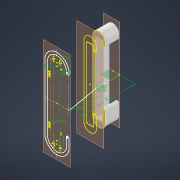
# Autodesk Inventor part: Top Part
Saved by Autodesk Inventor 2021.3 (Build 253353000, 353)
## iProperties
Created: 2021-07-04
Part Number: Top Part
Material: Generic
Document SubType Name: Modeling
Designer: trl121
Density: 1 g/cm^3
Appearance: Default
Author: trl121
Autodesk Inventor part; units mm, degrees
ref_plane "YZ Plane" through (0, 0, 0) normal (1, 0, 0) x (0, 1, 0)
ref_plane "XZ Plane" through (0, 0, 0) normal (0, 1, 0) x (-1, 0, 0)
ref_plane "XY Plane" through (0, 0, 0) normal (0, 0, 1) x (1, 0, 0)
ref_plane "Work Plane12" through (0, 0, 0) normal (0, 0, 1) x (1, 0, 0)
sketch "Sketch13" plane through (0, 0, 0) normal (0, 0, 1) x (1, 0, 0)
  line L0 (18.0369, 91.6315) -> (18.0369, 101.4813) projected
  arc A0 (12.9569, 86.5515) -> (18.0369, 91.6315) centre (12.9569, 91.6315) ccw projected
  arc A1 (10.4169, 87.8215) -> (11.6869, 86.5515) centre (11.6869, 87.8215) ccw projected
  line L1 (11.6869, 86.5515) -> (12.9569, 86.5515) projected
  line L2 (10.4169, 100.2113) -> (10.4169, 87.8215) projected
  arc A2 (18.0369, 101.4813) -> (-18.0369, 101.4813) centre (0, 101.4813) ccw projected
  arc A3 (10.4169, 100.2113) -> (9.1469, 101.4813) centre (9.1469, 100.2113) ccw projected
  line L3 (-9.1469, 101.4813) -> (9.1469, 101.4813) projected
  arc A4 (-9.1469, 101.4813) -> (-10.4169, 100.2113) centre (-9.1469, 100.2113) ccw projected
  line L4 (-10.4169, -100.2113) -> (-10.4169, 100.2113) projected
  line L5 (-18.0369, 101.4813) -> (-18.0369, 69.971) projected
  line L6 (-18.0369, 57.029) -> (-18.0369, -57.029) projected
  line L7 (-18.0369, -69.971) -> (-18.0369, -101.4813) projected
  arc A5 (-18.0369, -101.4813) -> (18.0369, -101.4813) centre (0, -101.4813) ccw projected
  line L8 (18.0369, -101.4813) -> (18.0369, -70.9285) projected
  arc A6 (18.0369, -70.9285) -> (12.9569, -65.8485) centre (12.9569, -70.9285) ccw projected
  line L9 (12.9569, -65.8485) -> (11.6869, -65.8485) projected
  arc A7 (11.6869, -65.8485) -> (10.4169, -67.1185) centre (11.6869, -67.1185) ccw projected
  line L10 (10.4169, -67.1185) -> (10.4169, -100.2113) projected
  arc A8 (9.1469, -101.4813) -> (10.4169, -100.2113) centre (9.1469, -100.2113) ccw projected
  line L11 (9.1469, -101.4813) -> (-9.1469, -101.4813) projected
  arc A9 (-10.4169, -100.2113) -> (-9.1469, -101.4813) centre (-9.1469, -100.2113) ccw projected
  line L12 (-18.0369, 69.971) -> (-18.0369, 57.029)
  line L13 (-18.0369, -57.029) -> (-18.0369, -69.971)
  line L14 (18.0369, 91.6315) -> (18.0369, -70.9285) construction
  point P0 (0, 0)
  constraints: 6 end point, 2 vertical, 1 collinear, 1 tangent
ref_plane "Work Plane4" through (-9.1469, 0, 0) normal (0, -1, 0) x (1, 0, 0)
sketch "Loft Sketch" plane through (-9.1469, 0, 0) normal (0, -1, 0) x (1, 0, 0)
  line L0 (27.1839, 65.45) -> (43.979, 160.7)
  line L1 (27.1839, 65.45) -> (27.1839, 40.05)
  point P0 (9.1469, 0)
  point P1 (27.1839, 0)
  point P2 (27.1839, 0)
  point P3 (27.1839, 0)
  dimension "d6" = 170
  dimension "d7" = 95.25
  dimension "d65" = 25.4
  dimension "d68" = 160.7
  constraints: 4 end point, 1 vertical, 1 vertical alignment
  measures "d6" angle of L0 L1
  measures "d7" vertical distance of L0.end L0.start
  measures "d65" distance of L0.start L1.end
  measures "d68" vertical distance of L0.end point (27.184, 0)
extrude "Extrusion6" add sketch "Sketch13" along normal up to surface (40.05 mm away)
sketch "Lower" plane through (0, 101.4813, 40.05) normal (0, 0, 1) x (1, 0, 0)
  line L0 (10.4169, -13.6598) -> (10.4169, -1.27) projected
  arc A0 (10.4169, -13.6598) -> (11.6869, -14.9298) centre (11.6869, -13.6598) ccw projected
  line L1 (12.9569, -14.9298) -> (11.6869, -14.9298) projected
  arc A1 (12.9569, -14.9298) -> (18.0369, -9.8498) centre (12.9569, -9.8498) ccw projected
  line L2 (18.0369, 0) -> (18.0369, -9.8498) projected
  arc A2 (18.0369, 0) -> (-18.0369, 0) centre (0, 0) ccw projected
  line L3 (-18.0369, -202.9627) -> (-18.0369, 0) projected
  arc A3 (-18.0369, -202.9627) -> (18.0369, -202.9627) centre (0, -202.9627) ccw projected
  line L4 (18.0369, -172.4098) -> (18.0369, -202.9627) projected
  arc A4 (18.0369, -172.4098) -> (12.9569, -167.3298) centre (12.9569, -172.4098) ccw projected
  line L5 (11.6869, -167.3298) -> (12.9569, -167.3298) projected
  arc A5 (11.6869, -167.3298) -> (10.4169, -168.5998) centre (11.6869, -168.5998) ccw projected
  line L6 (10.4169, -201.6927) -> (10.4169, -168.5998) projected
  arc A6 (9.1469, -202.9627) -> (10.4169, -201.6927) centre (9.1469, -201.6927) ccw projected
  line L7 (-9.1469, -202.9627) -> (9.1469, -202.9627) projected
  arc A7 (-10.4169, -201.6927) -> (-9.1469, -202.9627) centre (-9.1469, -201.6927) ccw projected
  line L8 (-10.4169, -1.27) -> (-10.4169, -201.6927) projected
  arc A8 (-9.1469, 0) -> (-10.4169, -1.27) centre (-9.1469, -1.27) ccw projected
  line L9 (9.1469, 0) -> (-9.1469, 0) projected
  arc A9 (10.4169, -1.27) -> (9.1469, 0) centre (9.1469, -1.27) ccw projected
  point P0 (0, -101.4813)
ref_plane "Mid Lof Plane" through (18.0369, 0, 65.45) normal (0, 0, 1) x (1, 0, 0)
sketch "Mid" plane through (18.0369, 0, 65.45) normal (0, 0, 1) x (1, 0, 0)
  line L0 (-7.62, 87.8215) -> (-7.62, 100.2113) projected
  arc A0 (-7.62, 87.8215) -> (-6.35, 86.5515) centre (-6.35, 87.8215) ccw projected
  line L1 (-5.08, 86.5515) -> (-6.35, 86.5515) projected
  arc A1 (-5.08, 86.5515) -> (0, 91.6315) centre (-5.08, 91.6315) ccw projected
  line L2 (0, 101.4813) -> (0, 91.6315) projected
  arc A2 (0, 101.4813) -> (-36.0739, 101.4813) centre (-18.0369, 101.4813) ccw projected
  line L3 (-36.0739, -101.4813) -> (-36.0739, 101.4813) projected
  arc A3 (-36.0739, -101.4813) -> (0, -101.4813) centre (-18.0369, -101.4813) ccw projected
  line L4 (0, -70.9285) -> (0, -101.4813) projected
  arc A4 (0, -70.9285) -> (-5.08, -65.8485) centre (-5.08, -70.9285) ccw projected
  line L5 (-6.35, -65.8485) -> (-5.08, -65.8485) projected
  arc A5 (-6.35, -65.8485) -> (-7.62, -67.1185) centre (-6.35, -67.1185) ccw projected
  line L6 (-7.62, -100.2113) -> (-7.62, -67.1185) projected
  arc A6 (-8.89, -101.4813) -> (-7.62, -100.2113) centre (-8.89, -100.2113) ccw projected
  line L7 (-27.1839, -101.4813) -> (-8.89, -101.4813) projected
  arc A7 (-28.4539, -100.2113) -> (-27.1839, -101.4813) centre (-27.1839, -100.2113) ccw projected
  line L8 (-28.4539, 100.2113) -> (-28.4539, -100.2113) projected
  arc A8 (-27.1839, 101.4813) -> (-28.4539, 100.2113) centre (-27.1839, 100.2113) ccw projected
  line L9 (-8.89, 101.4813) -> (-27.1839, 101.4813) projected
  arc A9 (-7.62, 100.2113) -> (-8.89, 101.4813) centre (-8.89, 100.2113) ccw projected
  point P0 (-18.0369, 0)
ref_plane "Work Plane5" through (34.8321, 0, 160.7) normal (0, 0, 1) x (1, 0, 0)
ref_plane "Work Plane7" through (0, 0, 0) normal (0, 0, 1) x (1, 0, 0)
sketch "Sketch6" plane through (34.8321, 0, 160.7) normal (0, 0, 1) x (1, 0, 0)
  line L0 (0, 92.3062) -> (0, 91.6315)
  line L1 (-62.0442, 92.3062) -> (-62.0442, 0)
  line L2 (-69.6642, 0) -> (-69.6642, 92.3062)
  line L3 (0, 91.6315) -> (0, 0) construction
  line L4 (-52.869, 0) -> (-45.249, 0) construction
  arc A0 (-34.8321, 119.5183) -> (-62.0442, 92.3062) centre (-34.8321, 92.3062) ccw
  arc A1 (-7.62, 92.3062) -> (-34.8321, 119.5183) centre (-34.8321, 92.3062) ccw
  line L5 (-7.62, 92.3062) -> (-7.62, 89.0915)
  arc A2 (-7.62, 89.0915) -> (-5.08, 86.5515) centre (-5.08, 89.0915) ccw
  line L6 (-5.08, 86.5515) -> (-5.08, 86.5515)
  arc A3 (-5.08, 86.5515) -> (0, 91.6315) centre (-5.08, 91.6315) ccw
  line L7 (-7.62, 90.6989) -> (0, 90.6989) construction
  line L8 (-69.6642, 0) -> (-62.0442, 0) construction
  arc A4 (0, 92.3062) -> (-69.6642, 92.3062) centre (-34.8321, 92.3062) ccw
  line L9 (0, 0) -> (-69.6642, 0) construction
  line L10 (0, -92.3062) -> (0, -70.9285)
  line L11 (-62.0442, -92.3062) -> (-62.0442, 0)
  line L12 (-69.6642, 0) -> (-69.6642, -92.3062)
  arc A5 (-62.0442, -92.3062) -> (-34.8321, -119.5183) centre (-34.8321, -92.3062) ccw
  arc A6 (-34.8321, -119.5183) -> (-7.62, -92.3062) centre (-34.8321, -92.3062) ccw
  line L13 (-7.62, -92.3062) -> (-7.62, -68.3885)
  arc A7 (-5.08, -65.8485) -> (-7.62, -68.3885) centre (-5.08, -68.3885) ccw
  line L14 (-5.08, -65.8485) -> (-5.08, -65.8485)
  arc A8 (0, -70.9285) -> (-5.08, -65.8485) centre (-5.08, -70.9285) ccw
  arc A9 (-69.6642, -92.3062) -> (0, -92.3062) centre (-34.8321, -92.3062) ccw
  arc A10 (-57.314, -56.6624) -> (-59.219, -57.7622) centre (-57.949, -57.7622) ccw construction
  line L15 (-59.219, -57.7622) -> (-59.219, -69.2378) construction
  arc A11 (-59.219, -69.2378) -> (-57.314, -70.3376) centre (-57.949, -69.2378) ccw construction
  line L16 (-57.314, -70.3376) -> (-54.774, -68.8712) construction
  arc A12 (-52.869, -69.971) -> (-54.774, -68.8712) centre (-54.139, -69.971) ccw construction
  line L17 (-52.869, -69.971) -> (-52.869, -101.4813) construction
  arc A13 (-52.869, -101.4813) -> (-16.7951, -101.4813) centre (-34.8321, -101.4813) ccw construction
  line L18 (-16.7951, -101.4813) -> (-16.7951, -70.9285) construction
  arc A14 (-16.7951, -70.9285) -> (-21.8751, -65.8485) centre (-21.8751, -70.9285) ccw construction
  line L19 (-21.8751, -65.8485) -> (-23.1451, -65.8485) construction
  arc A15 (-23.1451, -65.8485) -> (-24.4151, -67.1185) centre (-23.1451, -67.1185) ccw construction
  line L20 (-24.4151, -67.1185) -> (-24.4151, -100.2113) construction
  arc A16 (-25.6851, -101.4813) -> (-24.4151, -100.2113) centre (-25.6851, -100.2113) ccw construction
  line L21 (-25.6851, -101.4813) -> (-43.979, -101.4813) construction
  arc A17 (-45.249, -100.2113) -> (-43.979, -101.4813) centre (-43.979, -100.2113) ccw construction
  line L22 (-45.249, -100.2113) -> (-45.249, 100.2113) construction
  arc A18 (-43.979, 101.4813) -> (-45.249, 100.2113) centre (-43.979, 100.2113) ccw construction
  line L23 (-43.979, 101.4813) -> (-25.6851, 101.4813) construction
  arc A19 (-24.4151, 100.2113) -> (-25.6851, 101.4813) centre (-25.6851, 100.2113) ccw construction
  line L24 (-24.4151, 100.2113) -> (-24.4151, 87.8215) construction
  arc A20 (-24.4151, 87.8215) -> (-23.1451, 86.5515) centre (-23.1451, 87.8215) ccw construction
  line L25 (-23.1451, 86.5515) -> (-21.8751, 86.5515) construction
  arc A21 (-21.8751, 86.5515) -> (-16.7951, 91.6315) centre (-21.8751, 91.6315) ccw construction
  line L26 (-16.7951, 91.6315) -> (-16.7951, 101.4813) construction
  arc A22 (-16.7951, 101.4813) -> (-52.869, 101.4813) centre (-34.8321, 101.4813) ccw construction
  line L27 (-52.869, 101.4813) -> (-52.869, 69.971) construction
  arc A23 (-54.774, 68.8712) -> (-52.869, 69.971) centre (-54.139, 69.971) ccw construction
  line L28 (-54.774, 68.8712) -> (-57.314, 70.3376) construction
  arc A24 (-57.314, 70.3376) -> (-59.219, 69.2378) centre (-57.949, 69.2378) ccw construction
  line L29 (-59.219, 69.2378) -> (-59.219, 57.7622) construction
  arc A25 (-59.219, 57.7622) -> (-57.314, 56.6624) centre (-57.949, 57.7622) ccw construction
  line L30 (-57.314, 56.6624) -> (-54.774, 58.1288) construction
  arc A26 (-52.869, 57.029) -> (-54.774, 58.1288) centre (-54.139, 57.029) ccw construction
  line L31 (-52.869, 57.029) -> (-52.869, -57.029) construction
  arc A27 (-54.774, -58.1288) -> (-52.869, -57.029) centre (-54.139, -57.029) ccw construction
  line L32 (-54.774, -58.1288) -> (-57.314, -56.6624) construction
  line L33 (-42.4521, 102.7513) -> (-42.4521, 105.2913) construction
  arc A28 (-43.7221, 104.0213) -> (-42.4521, 105.2913) centre (-43.7221, 105.2913) ccw construction
  line L34 (-43.7221, 104.0213) -> (-47.5321, 104.0213) construction
  arc A29 (-48.8021, 105.2913) -> (-47.5321, 104.0213) centre (-47.5321, 105.2913) ccw construction
  line L35 (-48.8021, 105.2913) -> (-48.8021, 107.8313) construction
  arc A30 (-44.0396, 113.9797) -> (-48.8021, 107.8313) centre (-42.4521, 107.8313) ccw construction
  arc A31 (-42.4521, 112.75) -> (-44.0396, 113.9797) centre (-43.7221, 112.75) ccw construction
  line L36 (-42.4521, 112.75) -> (-42.4521, 109.1013) construction
  line L37 (-42.4521, 109.1013) -> (-27.2121, 109.1013) construction
  line L38 (-27.2121, 109.1013) -> (-27.2121, 112.75) construction
  arc A32 (-25.6246, 113.9797) -> (-27.2121, 112.75) centre (-25.9421, 112.75) ccw construction
  arc A33 (-20.8621, 107.8313) -> (-25.6246, 113.9797) centre (-27.2121, 107.8313) ccw construction
  line L39 (-20.8621, 107.8313) -> (-20.8621, 105.2913) construction
  arc A34 (-22.1321, 104.0213) -> (-20.8621, 105.2913) centre (-22.1321, 105.2913) ccw construction
  line L40 (-22.1321, 104.0213) -> (-25.9421, 104.0213) construction
  arc A35 (-27.2121, 105.2913) -> (-25.9421, 104.0213) centre (-25.9421, 105.2913) ccw construction
  line L41 (-27.2121, 105.2913) -> (-27.2121, 102.7513) construction
  line L42 (-27.2121, 102.7513) -> (-42.4521, 102.7513) construction
  line L43 (-27.2121, -109.1013) -> (-42.4521, -109.1013) construction
  line L44 (-42.4521, -109.1013) -> (-42.4521, -112.75) construction
  arc A36 (-44.0396, -113.9797) -> (-42.4521, -112.75) centre (-43.7221, -112.75) ccw construction
  arc A37 (-48.8021, -107.8313) -> (-44.0396, -113.9797) centre (-42.4521, -107.8313) ccw construction
  line L45 (-48.8021, -107.8313) -> (-48.8021, -105.2913) construction
  arc A38 (-47.5321, -104.0213) -> (-48.8021, -105.2913) centre (-47.5321, -105.2913) ccw construction
  line L46 (-47.5321, -104.0213) -> (-43.7221, -104.0213) construction
  arc A39 (-42.4521, -105.2913) -> (-43.7221, -104.0213) centre (-43.7221, -105.2913) ccw construction
  line L47 (-42.4521, -105.2913) -> (-42.4521, -102.7513) construction
  line L48 (-42.4521, -102.7513) -> (-27.2121, -102.7513) construction
  line L49 (-27.2121, -102.7513) -> (-27.2121, -105.2913) construction
  arc A40 (-25.9421, -104.0213) -> (-27.2121, -105.2913) centre (-25.9421, -105.2913) ccw construction
  line L50 (-25.9421, -104.0213) -> (-22.1321, -104.0213) construction
  arc A41 (-20.8621, -105.2913) -> (-22.1321, -104.0213) centre (-22.1321, -105.2913) ccw construction
  line L51 (-20.8621, -105.2913) -> (-20.8621, -107.8313) construction
  arc A42 (-25.6246, -113.9797) -> (-20.8621, -107.8313) centre (-27.2121, -107.8313) ccw construction
  arc A43 (-27.2121, -112.75) -> (-25.6246, -113.9797) centre (-25.9421, -112.75) ccw construction
  line L52 (-27.2121, -112.75) -> (-27.2121, -109.1013) construction
  line L53 (-24.4151, 94.0164) -> (-16.7951, 94.0164) construction
  line L54 (-45.249, 100.2113) -> (-52.869, 100.2113) construction
  line L55 (-62.0442, 92.3062) -> (-69.6642, 92.3062) construction
  line L56 (-57.949, -65.405) -> (-57.949, -61.595) projected
  arc A44 (-56.679, -60.325) -> (-57.949, -61.595) centre (-56.679, -61.595) ccw projected
  line L57 (-56.679, -60.325) -> (-55.409, -60.325) projected
  arc A45 (-54.139, -61.595) -> (-55.409, -60.325) centre (-55.409, -61.595) ccw projected
  line L58 (-54.139, -61.595) -> (-54.139, -65.405) projected
  arc A46 (-55.409, -66.675) -> (-54.139, -65.405) centre (-55.409, -65.405) ccw projected
  line L59 (-55.409, -66.675) -> (-56.679, -66.675) projected
  arc A47 (-57.949, -65.405) -> (-56.679, -66.675) centre (-56.679, -65.405) ccw projected
  line L60 (-57.949, 61.595) -> (-57.949, 65.405) projected
  arc A48 (-56.679, 66.675) -> (-57.949, 65.405) centre (-56.679, 65.405) ccw projected
  line L61 (-56.679, 66.675) -> (-55.409, 66.675) projected
  arc A49 (-54.139, 65.405) -> (-55.409, 66.675) centre (-55.409, 65.405) ccw projected
  line L62 (-54.139, 65.405) -> (-54.139, 61.595) projected
  arc A50 (-55.409, 60.325) -> (-54.139, 61.595) centre (-55.409, 61.595) ccw projected
  line L63 (-55.409, 60.325) -> (-56.679, 60.325) projected
  arc A51 (-57.949, 61.595) -> (-56.679, 60.325) centre (-56.679, 61.595) ccw projected
  point P0 (-34.8321, 0)
  point P1 (-34.8321, 127.1383)
  point P2 (-34.8321, -127.1383)
  dimension "d25" = 27.2121
  dimension "d26" = 27.2121
  dimension "d29" = 1.27
  dimension "d30" = 202.9627
  dimension "d31" = 9.1751
  constraints: 37 end point, 24 point on circle, 13 tangent, 10 centre point, 9 symmetric about line, 6 vertical, 5 perpendicular, 4 equal radius, 4 point on line, 3 collinear, 2 coincident, 2 horizontal, 2 midpoint, 2 parallel, 1 horizontal alignment, 5 other
  measures "d25" distance from line of L5 A22.centre
  measures "d26" distance from line of L1 A22.centre
  measures "d29" radius of A19
  measures "d30" distance between parallel lines of L21 L23
  measures "d31" distance between parallel lines of L5 L26
sketch "Sketch8" plane through (0, 101.4813, 0) normal (0, 0, -1) x (-1, 0, 0)
  arc A0 (19.9419, -170.3525) -> (18.0369, -171.4524) centre (19.3069, -171.4524) ccw projected
  line L0 (22.4819, -171.819) -> (19.9419, -170.3525) projected
  arc A1 (22.4819, -171.819) -> (24.3869, -170.7191) centre (23.1169, -170.7191) ccw projected
  line L1 (24.3869, -159.2435) -> (24.3869, -170.7191) projected
  arc A2 (24.3869, -159.2435) -> (22.4819, -158.1437) centre (23.1169, -159.2435) ccw projected
  line L2 (19.9419, -159.6102) -> (22.4819, -158.1437) projected
  arc A3 (18.0369, -158.5103) -> (19.9419, -159.6102) centre (19.3069, -158.5103) ccw projected
  line L3 (19.9419, -32.6102) -> (22.4819, -31.1437) projected
  arc A4 (18.0369, -31.5103) -> (19.9419, -32.6102) centre (19.3069, -31.5103) ccw projected
  arc A5 (24.3869, -32.2435) -> (22.4819, -31.1437) centre (23.1169, -32.2435) ccw projected
  line L4 (24.3869, -32.2435) -> (24.3869, -43.7191) projected
  arc A6 (19.9419, -43.3525) -> (18.0369, -44.4524) centre (19.3069, -44.4524) ccw projected
  line L5 (22.4819, -44.819) -> (19.9419, -43.3525) projected
  arc A7 (22.4819, -44.819) -> (24.3869, -43.7191) centre (23.1169, -43.7191) ccw projected
  line L6 (18.0369, -31.5103) -> (18.0369, -44.4524)
  line L7 (18.0369, 0) -> (18.0369, -202.9627) construction
  line L8 (18.0369, -171.4524) -> (18.0369, -158.5103)
  point P0 (0, -101.4813)
  constraints: 4 end point, 2 collinear
sketch "Sketch9" plane through (0, 101.4813, 0) normal (0, 0, -1) x (-1, 0, 0)
  line L0 (7.62, 7.62) -> (-7.62, 7.62) construction
  line L1 (7.62, 11.2687) -> (7.62, 7.62) construction
  arc A0 (9.2075, 12.4984) -> (7.62, 11.2687) centre (8.89, 11.2687) ccw construction
  arc A1 (13.97, 6.35) -> (9.2075, 12.4984) centre (7.62, 6.35) ccw construction
  line L2 (13.97, 3.81) -> (13.97, 6.35) construction
  arc A2 (12.7, 2.54) -> (13.97, 3.81) centre (12.7, 3.81) ccw construction
  line L3 (8.89, 2.54) -> (12.7, 2.54) construction
  line L4 (7.62, 1.27) -> (7.62, 3.81) construction
  line L5 (-7.62, 7.62) -> (-7.62, 11.2687) construction
  arc A3 (-7.62, 11.2687) -> (-9.2075, 12.4984) centre (-8.89, 11.2687) ccw construction
  arc A4 (-9.2075, 12.4984) -> (-13.97, 6.35) centre (-7.62, 6.35) ccw construction
  line L6 (-13.97, 6.35) -> (-13.97, 3.81) construction
  arc A5 (-13.97, 3.81) -> (-12.7, 2.54) centre (-12.7, 3.81) ccw construction
  line L7 (-12.7, 2.54) -> (-8.89, 2.54) construction
  line L8 (-7.62, 3.81) -> (-7.62, 1.27) construction
  line L9 (-7.62, 1.27) -> (7.62, 1.27) construction
  line L10 (-7.874, 2.286) -> (-12.7, 2.286)
  arc A6 (-14.224, 3.81) -> (-12.7, 2.286) centre (-12.7, 3.81) ccw
  line L11 (-14.224, 3.81) -> (-14.224, 6.35)
  arc A7 (-9.271, 12.7443) -> (-14.224, 6.35) centre (-7.62, 6.35) ccw
  arc A8 (-7.366, 11.2687) -> (-9.271, 12.7443) centre (-8.89, 11.2687) ccw
  line L12 (-7.366, 11.2687) -> (-7.366, 6.35)
  line L13 (7.366, 6.35) -> (7.366, 11.2687)
  arc A9 (9.271, 12.7443) -> (7.366, 11.2687) centre (8.89, 11.2687) ccw
  arc A10 (14.224, 6.35) -> (9.271, 12.7443) centre (7.62, 6.35) ccw
  line L14 (14.224, 6.35) -> (14.224, 3.81)
  arc A11 (12.7, 2.286) -> (14.224, 3.81) centre (12.7, 3.81) ccw
  line L15 (12.7, 2.286) -> (7.874, 2.286)
  line L16 (7.874, 2.286) -> (7.874, -0.254)
  line L17 (-7.874, -0.254) -> (-7.874, 2.286)
  line L18 (7.874, -0.254) -> (-7.874, -0.254)
  line L19 (9.1469, 0) -> (-9.1469, 0) construction
  line L20 (7.366, 6.35) -> (-7.366, 6.35)
  point P0 (0, -101.4813)
  dimension "d45" = 0.254
  dimension "d46" = 0.254
  dimension "d47" = 0.254
  dimension "d50" = 0.254
  dimension "d51" = 0.254
  dimension "d52" = 1.27
  constraints: 20 end point, 12 point on circle, 6 centre point, 1 horizontal, 1 parallel, 10 other
  measures "d45" distance between parallel lines of L16 L4
  measures "d46" distance between parallel lines of L8 L17
  measures "d47" distance between parallel lines of L18 L19
  measures "d50" distance between parallel lines of L13 L1
  measures "d51" distance between parallel lines of L12 L5
  measures "d52" distance between parallel lines of L0 L20
sketch "Sketch10" plane through (-7.366, 109.3553, 0) normal (-1, 0, 0) x (0, 0, 1)
  line L0 (-12.7, -1.016) -> (7.62, -1.524) construction
  line L1 (7.62, 1.016) -> (7.62, -1.524) construction
  line L2 (11.8332, -1.7226) -> (7.62, 1.016) construction
  line L3 (12.2002, -1.7226) -> (12.2002, -1.9766)
  line L4 (12.2002, -1.9766) -> (0, -1.9766)
  line L5 (0, -4.064) -> (0, -1.524) construction
  line L6 (12.2002, -1.7226) -> (7.42, 1.3845)
  line L7 (7.42, 1.3845) -> (7.42, -1.3189)
  line L8 (7.42, -1.3189) -> (0, 0.3094)
  line L9 (0, -1.9766) -> (0, 0.3094)
  point P0 (0, -109.3553)
  dimension "d53" = 0.254
  dimension "d57" = 0.2
  dimension "d58" = 2.286
  dimension "d59" = 0.2
  constraints: 12 end point, 3 point on line, 2 perpendicular, 1 horizontal alignment, 1 vertical, 1 other
  measures "d53" distance of L3.start L3.end
  measures "d57" distance between parallel lines of L6 L2
  measures "d58" distance of L4.end L9.end
  measures "d59" distance from line of L7.end L0
sketch "Sketch11" plane through (0, 101.4813, 0) normal (0, 0, -1) x (-1, 0, 0)
  arc A0 (19.3069, -39.8863) -> (20.5769, -41.1563) centre (20.5769, -39.8863) ccw construction
  line L0 (19.3069, -39.8863) -> (19.3069, -36.0763) construction
  arc A1 (20.5769, -34.8063) -> (19.3069, -36.0763) centre (20.5769, -36.0763) ccw construction
  line L1 (20.5769, -34.8063) -> (21.8469, -34.8063) construction
  arc A2 (23.1169, -36.0763) -> (21.8469, -34.8063) centre (21.8469, -36.0763) ccw construction
  line L2 (23.1169, -36.0763) -> (23.1169, -39.8863) construction
  arc A3 (21.8469, -41.1563) -> (23.1169, -39.8863) centre (21.8469, -39.8863) ccw construction
  line L3 (21.8469, -41.1563) -> (20.5769, -41.1563) construction
  arc A4 (23.1169, -163.0763) -> (21.8469, -161.8063) centre (21.8469, -163.0763) ccw construction
  line L4 (23.1169, -163.0763) -> (23.1169, -166.8863) construction
  arc A5 (21.8469, -168.1563) -> (23.1169, -166.8863) centre (21.8469, -166.8863) ccw construction
  line L5 (21.8469, -168.1563) -> (20.5769, -168.1563) construction
  arc A6 (19.3069, -166.8863) -> (20.5769, -168.1563) centre (20.5769, -166.8863) ccw construction
  line L6 (19.3069, -166.8863) -> (19.3069, -163.0763) construction
  arc A7 (20.5769, -161.8063) -> (19.3069, -163.0763) centre (20.5769, -163.0763) ccw construction
  line L7 (20.5769, -161.8063) -> (21.8469, -161.8063) construction
  line L8 (19.1069, -36.0763) -> (19.1069, -39.8863)
  arc A8 (19.1069, -39.8863) -> (20.5769, -41.3563) centre (20.5769, -39.8863) ccw
  line L9 (20.5769, -41.3563) -> (21.8469, -41.3563)
  arc A9 (21.8469, -41.3563) -> (23.3169, -39.8863) centre (21.8469, -39.8863) ccw
  line L10 (23.3169, -39.8863) -> (23.3169, -36.0763)
  arc A10 (23.3169, -36.0763) -> (21.8469, -34.6063) centre (21.8469, -36.0763) ccw
  line L11 (21.8469, -34.6063) -> (20.5769, -34.6063)
  arc A11 (20.5769, -34.6063) -> (19.1069, -36.0763) centre (20.5769, -36.0763) ccw
  line L12 (19.1069, -163.0763) -> (19.1069, -166.8863)
  arc A12 (19.1069, -166.8863) -> (20.5769, -168.3563) centre (20.5769, -166.8863) ccw
  line L13 (20.5769, -168.3563) -> (21.8469, -168.3563)
  arc A13 (21.8469, -168.3563) -> (23.3169, -166.8863) centre (21.8469, -166.8863) ccw
  line L14 (23.3169, -166.8863) -> (23.3169, -163.0763)
  arc A14 (23.3169, -163.0763) -> (21.8469, -161.6063) centre (21.8469, -163.0763) ccw
  line L15 (21.8469, -161.6063) -> (20.5769, -161.6063)
  arc A15 (20.5769, -161.6063) -> (19.1069, -163.0763) centre (20.5769, -163.0763) ccw
  point P0 (0, -101.4813)
  dimension "d60" = 0.2
  dimension "d61" = 0.2
  constraints: 16 end point, 16 point on circle, 8 centre point, 14 other
  measures "d60" distance between parallel lines of L0 L8
  measures "d61" distance between parallel lines of L6 L12
equation "\"d26\" = d25"
equation "\"d45\" = d50"
equation "\"d46\" = d50"
equation "\"d51\" = d50"
equation "\"d59\" = d57"
body "Solid2"
body "Solid3"
